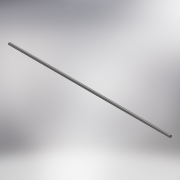
# Autodesk Inventor part: pipe
Saved by Autodesk Inventor 2018.2 (Build 222227000, 227)
## iProperties
Created: 2017-12-11
Part Number: pipe
Material: 鉄、可鍛鉄
Document SubType Name: Modeling
Designer: kuwano
Density: 7.15 g/cm^3
Appearance: 半つや出し
Mass: 213.924 g
Surface Area: 793.943 cm^2
Volume: 79.231 cm^3
Author: kuwano
Autodesk Inventor part; units mm, degrees
ref_plane "YZ Plane" through (0, 0, 0) normal (1, 0, 0) x (0, 1, 0)
ref_plane "XZ Plane" through (0, 0, 0) normal (0, 1, 0) x (-1, 0, 0)
ref_plane "XY Plane" through (0, 0, 0) normal (0, 0, 1) x (1, 0, 0)
sketch "スケッチ1" plane through (0, 0, 0) normal (1, 0, 0) x (0, 1, 0)
  circle A0 centre (0, 0) radius 7.5
  dimension "d0" = 15
  constraints: 1 centre point, 1 coincident
  measures "d0" diameter of A0
extrude "押し出し1" add sketch "スケッチ1" along normal mid plane 950
shell "シェル1" thickness 2 removed faces 2 at (475, 1.2064, -0.2974) at (-475, 1.2064, -0.2974)
thread "ねじ1" size "M11x1.5" class "6H" standard "ANSI Metric M Profile" length 20
thread "ねじ2" size "M11x1.5" class "6H" standard "ANSI Metric M Profile" length 10
